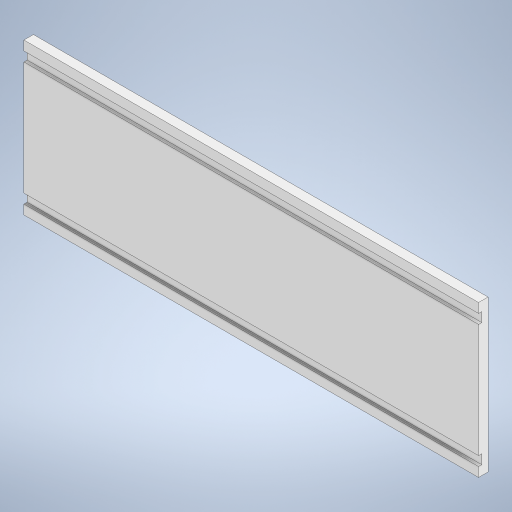
# Autodesk Inventor part: MS_R_Front_bottom_yellow_v3
Saved by Autodesk Inventor 2024 (Build 280153000, 153)
## iProperties
Created: 2024-02-15
Part Number: MS_R_Front_bottom_yellow_v3
Material: Generic
Document SubType Name: Modeling
Designer: LKLM
Density: 1 g/cm^3
Appearance: White
Author: LKLM
Autodesk Inventor part; units mm, degrees
ref_plane "YZ Plane" through (0, 0, 0) normal (1, 0, 0) x (0, 1, 0)
ref_plane "XZ Plane" through (0, 0, 0) normal (0, 1, 0) x (-1, 0, 0)
ref_plane "XY Plane" through (0, 0, 0) normal (0, 0, 1) x (1, 0, 0)
sketch "Sketch1" plane through (0, 0, 0) normal (0, 0, 1) x (1, 0, 0)
  line L0 (0, 0) -> (-72, 0)
  line L1 (0, 24) -> (0, 0)
  line L2 (0, 0) -> (0, 24) construction
  line L3 (-72, 24) -> (0, 24)
  line L4 (-72, 0) -> (-72, 24)
  point P0 (0, 0)
  point P1 (-137.4598, 47.0487)
  dimension "d3" = 0
  dimension "d4" = 0
  dimension "d8" = 24
  constraints: 10 end point, 1 horizontal, 1 parallel, 1 perpendicular
  measures "d3" distance from line of L0 point (0, 0)
  measures "d4" distance from line of L1 point (0, 0)
  measures "d8" distance of L1.start L1.end
extrude "Extrusion2" add sketch "Sketch1" along normal blind 1.5
sketch "Sketch2" plane through (0, 0, 1.5) normal (0, 0, 1) x (1, 0, 0)
  line L0 (0, 0) -> (0, 24) projected
  line L1 (0, 1.5) -> (-72, 1.5)
  line L2 (-72, 1.5) -> (-72, 3)
  line L3 (-72, 3) -> (0, 3)
  line L4 (0, 3) -> (0, 1.5)
  line L5 (0, 22.5) -> (-72, 22.5)
  line L6 (-72, 22.5) -> (-72, 21)
  line L7 (-72, 21) -> (0, 21)
  line L8 (0, 21) -> (0, 22.5)
  point P0 (0, 3)
  point P1 (0, 21)
  dimension "d59" = 72
  dimension "d60" = 1.5
  dimension "d61" = 1.5
  constraints: 16 end point, 4 parallel, 3 point on line, 2 horizontal, 2 perpendicular
  measures "d59" distance of L2.end L3.end
  measures "d60" distance of L1.end L2.end
  measures "d61" distance of L6.end L5.end
extrude "Extrusion3" cut sketch "Sketch2" against normal blind 0.5
body "Solid2"
